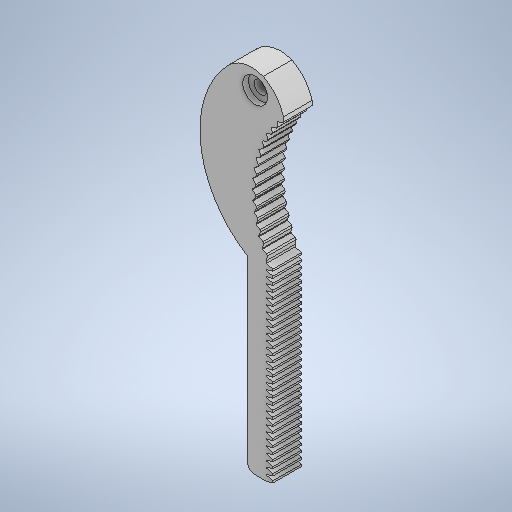
# Autodesk Inventor part: gripper part
Saved by Autodesk Inventor 2026.1 (Build 301233000, 233)
## iProperties
Created: 2025-10-10
Part Number: gripper part
Material: Generic
Document SubType Name: Modeling
Designer: shahn
Density: 1 g/cm^3
Appearance: Default
Author: shahn
Autodesk Inventor part; units mm, degrees
ref_plane "YZ Plane" through (0, 0, 0) normal (1, 0, 0) x (0, 1, 0)
ref_plane "XZ Plane" through (0, 0, 0) normal (0, 1, 0) x (-1, 0, 0)
ref_plane "XY Plane" through (0, 0, 0) normal (0, 0, 1) x (1, 0, 0)
sketch "Sketch1" plane through (0, 0, 0) normal (0, 0, 1) x (1, 0, 0)
  line L0 (23.6777, -10) -> (18.6777, -10)
  line L1 (18.6777, -10) -> (18.6777, 40)
  arc A0 (18.6122, 79.9999) -> (18.6777, 40) centre (33.6449, 60.0245) ccw
  arc A1 (23.6777, 40.0089) -> (22.8328, 79.9999) centre (8.2586, 59.6876) ccw
  arc A2 (22.8328, 79.9999) -> (18.6122, 79.9999) centre (20.7225, 77.1958) ccw
  line L2 (23.6777, 40.0089) -> (23.6777, -10)
  line L3 (23.6777, -10) -> (25.368, -9.5471)
  line L4 (23.6777, -10) -> (25.4277, -10) construction
  line L5 (25.368, -9.5471) -> (25.368, -9.0471)
  line L6 (25.368, -9.0471) -> (23.6777, -8.5941)
  line L7 (25.368, -7.4471) -> (23.6777, -6.9941)
  line L8 (25.368, -7.9471) -> (25.368, -7.4471)
  line L9 (23.6777, -8.4) -> (25.368, -7.9471)
  line L10 (25.368, -5.8471) -> (23.6777, -5.3941)
  line L11 (25.368, -6.3471) -> (25.368, -5.8471)
  line L12 (23.6777, -6.8) -> (25.368, -6.3471)
  line L13 (25.368, -4.2471) -> (23.6777, -3.7941)
  line L14 (25.368, -4.7471) -> (25.368, -4.2471)
  line L15 (23.6777, -5.2) -> (25.368, -4.7471)
  line L16 (25.368, -2.6471) -> (23.6777, -2.1941)
  line L17 (25.368, -3.1471) -> (25.368, -2.6471)
  line L18 (23.6777, -3.6) -> (25.368, -3.1471)
  line L19 (25.368, -1.0471) -> (23.6777, -0.5941)
  line L20 (25.368, -1.5471) -> (25.368, -1.0471)
  line L21 (23.6777, -2) -> (25.368, -1.5471)
  line L22 (25.368, 0.5529) -> (23.6777, 1.0059)
  line L23 (25.368, 0.0529) -> (25.368, 0.5529)
  line L24 (23.6777, -0.4) -> (25.368, 0.0529)
  line L25 (25.368, 2.1529) -> (23.6777, 2.6059)
  line L26 (25.368, 1.6529) -> (25.368, 2.1529)
  line L27 (23.6777, 1.2) -> (25.368, 1.6529)
  line L28 (25.368, 3.7529) -> (23.6777, 4.2059)
  line L29 (25.368, 3.2529) -> (25.368, 3.7529)
  line L30 (23.6777, 2.8) -> (25.368, 3.2529)
  line L31 (25.368, 5.3529) -> (23.6777, 5.8059)
  line L32 (25.368, 4.8529) -> (25.368, 5.3529)
  line L33 (23.6777, 4.4) -> (25.368, 4.8529)
  line L34 (25.368, 6.9529) -> (23.6777, 7.4059)
  line L35 (25.368, 6.4529) -> (25.368, 6.9529)
  line L36 (23.6777, 6) -> (25.368, 6.4529)
  line L37 (25.368, 8.5529) -> (23.6777, 9.0059)
  line L38 (25.368, 8.0529) -> (25.368, 8.5529)
  line L39 (23.6777, 7.6) -> (25.368, 8.0529)
  line L40 (25.368, 10.1529) -> (23.6777, 10.6059)
  line L41 (25.368, 9.6529) -> (25.368, 10.1529)
  line L42 (23.6777, 9.2) -> (25.368, 9.6529)
  line L43 (25.368, 11.7529) -> (23.6777, 12.2059)
  line L44 (25.368, 11.2529) -> (25.368, 11.7529)
  line L45 (23.6777, 10.8) -> (25.368, 11.2529)
  line L46 (25.368, 13.3529) -> (23.6777, 13.8059)
  line L47 (25.368, 12.8529) -> (25.368, 13.3529)
  line L48 (23.6777, 12.4) -> (25.368, 12.8529)
  line L49 (25.368, 14.9529) -> (23.6777, 15.4059)
  line L50 (25.368, 14.4529) -> (25.368, 14.9529)
  line L51 (23.6777, 14) -> (25.368, 14.4529)
  line L52 (25.368, 16.5529) -> (23.6777, 17.0059)
  line L53 (25.368, 16.0529) -> (25.368, 16.5529)
  line L54 (23.6777, 15.6) -> (25.368, 16.0529)
  line L55 (25.368, 18.1529) -> (23.6777, 18.6059)
  line L56 (25.368, 17.6529) -> (25.368, 18.1529)
  line L57 (23.6777, 17.2) -> (25.368, 17.6529)
  line L58 (25.368, 19.7529) -> (23.6777, 20.2059)
  line L59 (25.368, 19.2529) -> (25.368, 19.7529)
  line L60 (23.6777, 18.8) -> (25.368, 19.2529)
  line L61 (25.368, 21.3529) -> (23.6777, 21.8059)
  line L62 (25.368, 20.8529) -> (25.368, 21.3529)
  line L63 (23.6777, 20.4) -> (25.368, 20.8529)
  line L64 (25.368, 22.9529) -> (23.6777, 23.4059)
  line L65 (25.368, 22.4529) -> (25.368, 22.9529)
  line L66 (23.6777, 22) -> (25.368, 22.4529)
  line L67 (25.368, 24.5529) -> (23.6777, 25.0059)
  line L68 (25.368, 24.0529) -> (25.368, 24.5529)
  line L69 (23.6777, 23.6) -> (25.368, 24.0529)
  line L70 (25.368, 26.1529) -> (23.6777, 26.6059)
  line L71 (25.368, 25.6529) -> (25.368, 26.1529)
  line L72 (23.6777, 25.2) -> (25.368, 25.6529)
  line L73 (25.368, 27.7529) -> (23.6777, 28.2059)
  line L74 (25.368, 27.2529) -> (25.368, 27.7529)
  line L75 (23.6777, 26.8) -> (25.368, 27.2529)
  line L76 (25.368, 29.3529) -> (23.6777, 29.8059)
  line L77 (25.368, 28.8529) -> (25.368, 29.3529)
  line L78 (23.6777, 28.4) -> (25.368, 28.8529)
  line L79 (25.368, 30.9529) -> (23.6777, 31.4059)
  line L80 (25.368, 30.4529) -> (25.368, 30.9529)
  line L81 (23.6777, 30) -> (25.368, 30.4529)
  line L82 (25.368, 32.5529) -> (23.6777, 33.0059)
  line L83 (25.368, 32.0529) -> (25.368, 32.5529)
  line L84 (23.6777, 31.6) -> (25.368, 32.0529)
  line L85 (25.368, 34.1529) -> (23.6777, 34.6059)
  line L86 (25.368, 33.6529) -> (25.368, 34.1529)
  line L87 (23.6777, 33.2) -> (25.368, 33.6529)
  line L88 (25.368, 35.7529) -> (23.6777, 36.2059)
  line L89 (25.368, 35.2529) -> (25.368, 35.7529)
  line L90 (23.6777, 34.8) -> (25.368, 35.2529)
  line L91 (25.368, 37.3529) -> (23.6777, 37.8059)
  line L92 (25.368, 36.8529) -> (25.368, 37.3529)
  line L93 (23.6777, 36.4) -> (25.368, 36.8529)
  line L94 (25.368, 38.9529) -> (23.6777, 39.4059)
  line L95 (25.368, 38.4529) -> (25.368, 38.9529)
  line L96 (23.6777, 38) -> (25.368, 38.4529)
  point P0 (0, 0)
  point P1 (20.7225, 80.7053)
  point P2 (33.253, 60.2156)
  point P3 (25.4277, -8.4)
  point P4 (25.4277, -6.8)
  point P5 (25.4277, -5.2)
  point P6 (25.4277, -3.6)
  point P7 (25.4277, -2)
  point P8 (25.4277, -0.4)
  point P9 (25.4277, 1.2)
  point P10 (25.4277, 2.8)
  point P11 (25.4277, 4.4)
  point P12 (25.4277, 6)
  point P13 (25.4277, 7.6)
  point P14 (25.4277, 9.2)
  point P15 (25.4277, 10.8)
  point P16 (25.4277, 12.4)
  point P17 (25.4277, 14)
  point P18 (25.4277, 15.6)
  point P19 (25.4277, 17.2)
  point P20 (25.4277, 18.8)
  point P21 (25.4277, 20.4)
  point P22 (25.4277, 22)
  point P23 (25.4277, 23.6)
  point P24 (25.4277, 25.2)
  point P25 (25.4277, 26.8)
  point P26 (23.6777, 25.2)
  point P27 (23.6777, 22)
  point P28 (23.6777, 20.2059)
  point P29 (23.6777, 18.8)
  point P30 (23.6777, 12.4)
  point P31 (23.6777, 10.6059)
  point P32 (23.6777, 9.0059)
  point P33 (23.6777, 7.6)
  point P34 (23.6777, 7.4059)
  point P35 (23.6777, 6)
  point P36 (23.6777, 5.8059)
  point P37 (23.6777, 4.4)
  point P38 (23.6777, 4.2059)
  point P39 (23.6777, 2.8)
  point P40 (23.6777, 2.6059)
  point P41 (23.6777, 1.2)
  point P42 (23.6777, 1.0059)
  point P43 (23.6777, -0.4)
  point P44 (23.6777, -0.5941)
  point P45 (23.6777, -2)
  point P46 (23.6777, -2.1941)
  point P47 (23.6777, -3.6)
  point P48 (23.6777, -3.7941)
  point P49 (23.6777, -5.2)
  point P50 (23.6777, -5.3941)
  point P51 (23.6777, -6.8)
  point P52 (23.6777, -8.4)
  point P53 (25.4277, 28.4)
  point P54 (25.4277, 30)
  point P55 (25.4277, 31.6)
  point P56 (25.4277, 33.2)
  point P57 (25.4277, 34.8)
  point P58 (25.4277, 36.4)
  point P59 (25.4277, 38)
  dimension "d38" = 5
  dimension "d39" = 50
  dimension "d40" = 40
  dimension "d41" = 25
  dimension "d42" = 40
  dimension "d43" = 25
  dimension "d52" = 3.5095
  dimension "d53" = 40
  dimension "d54" = 59.6876
  dimension "d55" = 33.253
  dimension "d56" = 80.7053
  dimension "d116" = 1.75
  dimension "d117" = 15
  dimension "d118" = 0.5
  dimension "d119" = 105
  dimension "d122" = 1.6
  constraints: 192 end point, 150 vertical alignment, 60 parallel, 30 collinear, 8 point on circle, 3 centre point, 2 horizontal, 1 equal length, 1 perpendicular, 1 tangent, 1 vertical, 4 other
  measures "d38" distance of L0.start L0.end
  measures "d39" distance of L0.end L1.end
  measures "d40" distance of L1.end A0.start
  measures "d41" radius of A0
  measures "d42" distance of A1.start A1.end
  measures "d43" radius of A1
  measures "d52" distance of point (20.722, 80.705) A2.centre
  measures "d53" vertical distance of point (0, 0) L1.end
  measures "d54" vertical distance of point (0, 0) A1.centre
  measures "d55" horizontal distance of point (33.253, 60.216) point (0, 0)
  measures "d56" vertical distance of point (0, 0) point (20.722, 80.705)
  measures "d116" distance of L0.start L3.end
  measures "d117" angle of L4 L3
  measures "d118" distance of L3.end L5.end
  measures "d119" angle of L6 L5
  measures "d122" distance of L6.end L7.end
extrude "Extrusion5" add sketch "Sketch1" along normal blind 7.5
sketch "Sketch2" plane through (0, 0, 7.5) normal (0, 0, 1) x (1, 0, 0)
  arc A0 (23.6777, 40.0089) -> (22.8328, 79.9999) centre (8.2586, 59.6876) ccw projected
  line L0 (23.6777, 29.1814) -> (23.6777, 40.0089) projected
  arc A1 (28.1285, 74.8594) -> (23.6777, 40.0089) centre (50.026, 54.3534) ccw
  line L1 (23.6777, 40.0089) -> (23.9338, 41.1812)
  line L2 (23.9338, 41.1812) -> (23.7453, 41.6443)
  line L3 (23.7453, 41.6443) -> (22.6387, 42.1085)
  line L4 (22.7739, 43.8884) -> (21.71, 44.4435)
  line L5 (22.9229, 43.4111) -> (22.7739, 43.8884)
  line L6 (22.5696, 42.2643) -> (22.9229, 43.4111)
  line L7 (21.9937, 46.2058) -> (20.98, 46.8481)
  line L8 (22.1022, 45.7177) -> (21.9937, 46.2058)
  line L9 (21.6542, 44.6045) -> (22.1022, 45.7177)
  line L10 (21.4101, 48.5804) -> (20.4538, 49.3053)
  line L11 (21.4775, 48.085) -> (21.4101, 48.5804)
  line L12 (20.9378, 47.0132) -> (21.4775, 48.085)
  line L13 (21.0274, 50.9956) -> (20.1351, 51.7979)
  line L14 (21.053, 50.4962) -> (21.0274, 50.9956)
  line L15 (20.4256, 49.4733) -> (21.053, 50.4962)
  line L16 (20.8481, 53.4342) -> (20.0261, 54.3084)
  line L17 (20.8319, 52.9345) -> (20.8481, 53.4342)
  line L18 (20.121, 51.9677) -> (20.8319, 52.9345)
  line L19 (20.8735, 55.8794) -> (20.1275, 56.8193)
  line L20 (20.8155, 55.3827) -> (20.8735, 55.8794)
  line L21 (20.0263, 54.4788) -> (20.8155, 55.3827)
  line L22 (21.1035, 58.3138) -> (20.4388, 59.3129)
  line L23 (21.0042, 57.8238) -> (21.1035, 58.3138)
  line L24 (20.142, 56.9891) -> (21.0042, 57.8238)
  line L25 (21.5364, 60.7204) -> (20.9577, 61.7716)
  line L26 (21.3964, 60.2404) -> (21.5364, 60.7204)
  line L27 (20.4674, 59.4808) -> (21.3964, 60.2404)
  line L28 (22.1693, 63.0824) -> (21.6805, 64.1783)
  line L29 (21.9896, 62.6158) -> (22.1693, 63.0824)
  line L30 (21.0003, 61.9366) -> (21.9896, 62.6158)
  line L31 (22.9975, 65.3831) -> (22.6022, 66.5161)
  line L32 (22.7794, 64.9332) -> (22.9975, 65.3831)
  line L33 (21.7367, 64.3392) -> (22.7794, 64.9332)
  line L34 (24.0154, 67.6064) -> (23.7163, 68.7686)
  line L35 (23.7604, 67.1764) -> (24.0154, 67.6064)
  line L36 (22.6717, 66.6717) -> (23.7604, 67.1764)
  line L37 (25.2158, 69.7368) -> (25.015, 70.9199)
  line L38 (24.9257, 69.3295) -> (25.2158, 69.7368)
  line L39 (23.7986, 68.9178) -> (24.9257, 69.3295)
  line L40 (26.5903, 71.7592) -> (26.4892, 72.9549)
  line L41 (26.2671, 71.3777) -> (26.5903, 71.7592)
  line L42 (25.1095, 71.0616) -> (26.2671, 71.3777)
  line L43 (28.1292, 73.6595) -> (28.1285, 74.8595)
  line L44 (27.7753, 73.3063) -> (28.1292, 73.6595)
  line L45 (26.5952, 73.0883) -> (27.7753, 73.3063)
  arc A2 (22.8328, 79.9999) -> (18.6122, 79.9999) centre (20.7225, 77.1958) ccw projected
  point P0 (0, 0)
  point P1 (20.7225, 80.7053)
  point P2 (28.1285, 74.8594)
  dimension "d59" = 30
  dimension "d60" = 1.2
  dimension "d61" = 0.5
  dimension "d62" = 1.2
  dimension "d63" = 134.9
  dimension "d64" = 145.535
  dimension "d67" = 67.21
  dimension "d69" = 7.406
  constraints: 90 end point, 2 point on circle, 104 other
  measures "d60" distance of L0.end L1.end
  measures "d61" distance of L1.end L2.end
  measures "d62" distance of L2.end L3.end
  measures "d63" angle of L2 L3
  measures "d64" angle of L1 L2
  measures "d69" horizontal distance of point (20.722, 80.705) L43.end
extrude "Extrusion6" cut sketch "Sketch2" against normal blind 10 contours L1 L2 L3 A1 L6 L5 L4 L9 L8 L7 L12 L11 L10 L15 L14 L13 L18 L17 L16 L21 L20 L19 L24 L23 L22 L27 L26 L25 L30 L29 L28 L33 L32 L31 L36 L35 L34 L39 L38 L37 L42 L41 L40 L45 L44 L43 A0
fillet "Fillet3" radius 2 1 edges at (18.6777, -10, 3.75)
fillet "Fillet4" radius 2 1 edges at (18.6777, 40, 3.75)
sketch "Sketch3" plane through (0, 0, 7.5) normal (0, 0, 1) x (1, 0, 0)
  circle A0 centre (20.7225, 77.1958) radius 1.7
  arc A1 (22.8328, 79.9999) -> (18.6122, 79.9999) centre (20.7225, 77.1958) ccw projected
  point P0 (0, 0)
  dimension "d74" = 3.4
  constraints: 1 centre point, 1 concentric
  measures "d74" diameter of A0
extrude "Extrusion7" cut sketch "Sketch3" against normal blind 10
sketch "Sketch4" plane through (0, 0, 7.5) normal (0, 0, 1) x (1, 0, 0)
  circle A0 centre (20.7225, 77.1958) radius 1.7 projected
  circle A1 centre (20.7225, 77.1958) radius 3.25
  point P0 (0, 0)
  dimension "d77" = 6.5
  constraints: 1 centre point, 1 coincident
  measures "d77" diameter of A1
sketch "Sketch5" plane through (0, 0, 0) normal (0, 0, -1) x (-1, 0, 0)
  circle A0 centre (-20.7225, 77.1958) radius 1.7 projected
  circle A1 centre (-20.7225, 77.1958) radius 3.25
  point P0 (0, 0)
  dimension "d78" = 6.5
  constraints: 1 centre point, 1 coincident
  measures "d78" diameter of A1
extrude "Extrusion8" cut sketch "Sketch5" against normal blind 1.5
extrude "Extrusion9" cut sketch "Sketch4" against normal blind 1.5
sketch "Sketch6" plane through (0, 0, 7.5) normal (0, 0, 1) x (1, 0, 0)
  arc A0 (28.1285, 74.8594) -> (22.8328, 79.9999) centre (8.2586, 59.6876) ccw projected
  arc A1 (28.1285, 74.8594) -> (22.8328, 81.3776) centre (18.0299, 72.0651) ccw
  arc A2 (18.6122, 79.9999) -> (17.9345, 40.5776) centre (33.6449, 60.0245) ccw projected
  arc A3 (13.6783, 79.3399) -> (18.6777, 38.6006) centre (32.6457, 60.9911) ccw
  arc A4 (22.8328, 81.3776) -> (13.6783, 79.3399) centre (19.8006, 73.4172) ccw
  line L0 (18.6777, 39.0218) -> (18.6777, -8) projected
  arc A5 (18.6777, 39.0218) -> (17.9345, 40.5776) centre (16.6777, 39.0218) ccw projected
  arc A6 (22.8328, 79.9999) -> (18.6122, 79.9999) centre (20.7225, 77.1958) ccw projected
  point P0 (0, 0)
  dimension "d83" = 10.4781
  dimension "d84" = 8.5183
  dimension "d85" = 26.3902
  dimension "d86" = 38.6006
  dimension "d87" = 79.3399
  dimension "d88" = 81.3776
  constraints: 6 point on circle, 3 centre point, 2 tangent, 1 point on line
  measures "d83" radius of A1
  measures "d84" radius of A4
  measures "d85" radius of A3
  measures "d86" vertical distance of point (0, 0) A3.end
  measures "d87" vertical distance of point (0, 0) A3.start
  measures "d88" vertical distance of point (0, 0) A1.end
extrude "Extrusion10" add sketch "Sketch6" against normal blind 7.5
body "Solid5"
